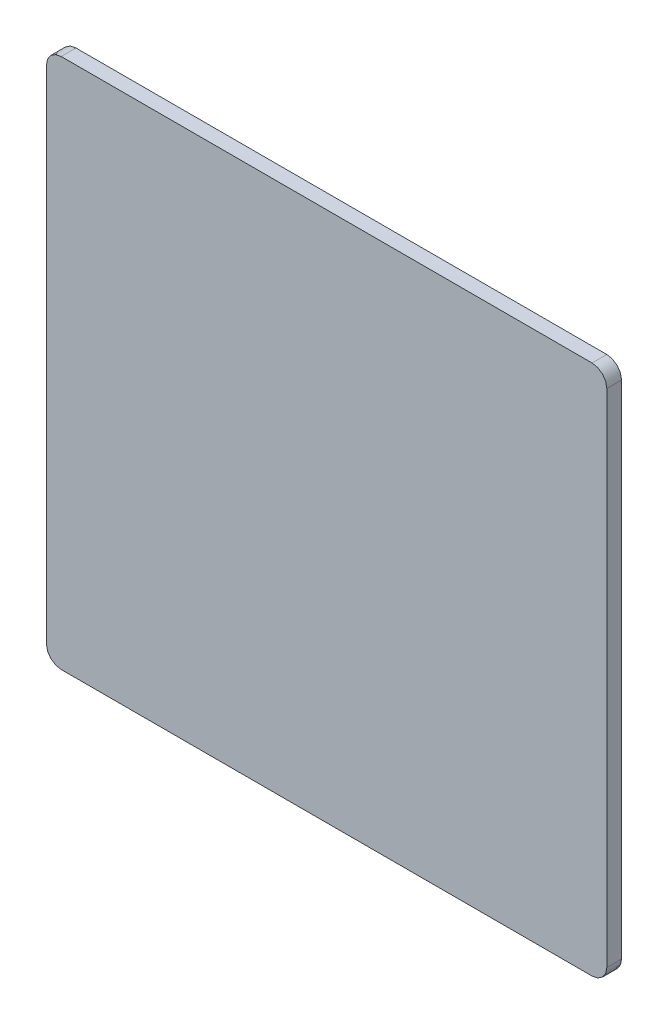
# Autodesk Inventor part: SitzflächeGlas
Saved by Autodesk Inventor 2018 (Build 220112000, 112)
## iProperties
Created: 2019-03-25
Part Number: SitzflächeGlas
Material: Glas
Document SubType Name: Modeling
Designer: DerLobre
Density: 2.18 g/cm^3
Appearance: Klar
Author: DerLobre
Autodesk Inventor part; units mm, degrees
ref_plane "YZ Plane" through (0, 0, 0) normal (1, 0, 0) x (0, 1, 0)
ref_plane "XZ Plane" through (0, 0, 0) normal (0, 1, 0) x (-1, 0, 0)
ref_plane "XY Plane" through (0, 0, 0) normal (0, 0, 1) x (1, 0, 0)
ref_plane "Arbeitsebene1" through (0, -25, 0) normal (0, 0, 1) x (1, 0, 0)
sketch "Skizze1" plane through (0, -25, 0) normal (0, 0, 1) x (1, 0, 0)
  arc A0 (-170, 170) -> (-180, 160) centre (-170, 160) ccw projected
  line L0 (-170, 170) -> (170, 170) projected
  arc A1 (180, 160) -> (170, 170) centre (170, 160) ccw projected
  line L1 (180, 160) -> (180, -160) projected
  line L2 (-180, -160) -> (-180, 160) projected
  arc A2 (-180, 180) -> (-190, 170) centre (-180, 170) ccw projected
  line L3 (-190, -170) -> (-190, 170) projected
  arc A3 (-190, -170) -> (-180, -180) centre (-180, -170) ccw projected
  arc A4 (180, -180) -> (190, -170) centre (180, -170) ccw projected
  line L4 (190, 170) -> (190, -170) projected
  arc A5 (190, 170) -> (180, 180) centre (180, 170) ccw projected
  line L5 (180, 165) -> (-180, 165)
  line L6 (-190, 155) -> (-190, -155)
  line L7 (-180, -165) -> (180, -165)
  line L8 (190, -155) -> (190, 155)
  arc A6 (-190, -155) -> (-180, -165) centre (-180, -155) ccw
  arc A7 (-180, 165) -> (-190, 155) centre (-180, 155) ccw
  arc A8 (190, 155) -> (180, 165) centre (180, 155) ccw
  arc A9 (180, -165) -> (190, -155) centre (180, -155) ccw
  arc A10 (170, -170) -> (180, -160) centre (170, -160) ccw projected
  line L9 (170, -170) -> (-170, -170) projected
  arc A11 (-180, -160) -> (-170, -170) centre (-170, -160) ccw projected
  line L10 (-180, 180) -> (180, 180) projected
  line L11 (180, -180) -> (-180, -180) projected
  point P0 (0, 25)
  dimension "d0" = 10
  constraints: 8 end point, 8 point on circle, 8 tangent, 4 centre point, 3 equal radius, 2 parallel, 1 horizontal, 1 perpendicular
  measures "d0" radius of A6
extrude "Extrusion1" add sketch "Skizze1" along normal blind 10
